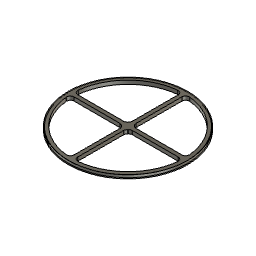
wheel v6 (Autodesk Fusion 360 design; units mm, degrees)
Autodesk Fusion 360 part; units mm, degrees
sketch "Sketch1" plane through (0, 0, 0) normal (0, 0, 1) x (1, 0, 0)
  circle A0 centre (0, 0) radius 41.275
  circle A1 centre (0, 0) radius 38.735
  circle A2 centre (0, 0) radius 3.175
  dimension "d1" = 82.55
  dimension "d2" = 77.47
  dimension "d5" = 6.35
  constraint coincident A0.centre A1.centre
  measures "d1" diameter of A0
  measures "d2" diameter of A1
  measures "d5" diameter of A2
extrude "Extrude1" add sketch "Sketch1" along normal blind 2.54 makes body 1 at (41.2237, -2.0574, 1.6933) makes body 2 at (3.1711, -0.1583, 1.6933)
sketch "Sketch4" plane through (0, 0, 0) normal (0, 0, 1) x (1, 0, 0)
  line L0 (-1.27, 39.37) -> (1.27, 39.37)
  line L1 (1.27, 39.37) -> (1.27, 1.27)
  line L2 (1.27, 1.27) -> (-1.27, 1.27)
  line L3 (-1.27, 1.27) -> (-1.27, 39.37)
  dimension "d12" = 2.54
  dimension "d13" = 1.27
  dimension "d14" = 38.1
  dimension "d15" = 1.27
  constraint horizontal L0
  constraint vertical L1
  constraint horizontal L2
  constraint vertical L3
  measures "d12" distance of L1.end L2.end
  measures "d13" horizontal distance of origin L1.end
  measures "d14" distance of L0.end L1.end
  measures "d15" vertical distance of origin L2.end
extrude "Extrude3" add sketch "Sketch4" along normal blind 2.54 separate body makes body 3
pattern_circular "C-Pattern1" count 4 over 360 about axis through (0, 0, 1.75) along (0, 0, 1) of bodies 3 makes body 4 at (-26.67, 1.27, 0.8467) makes body 5 at (-1.27, -26.67, 0.8467) makes body 6 at (26.67, -1.27, 0.8467)
combine "Combine1" operation add target body 3 tool bodies 1 2 6 5 4
fillet "Fillet1" radius 2.54 8 edges at (2.9099, 1.27, 1.27) (1.27, 2.9099, 1.27) (-1.27, 2.9099, 1.27) (-2.9099, 1.27, 1.27) (-2.9099, -1.27, 1.27) (-1.27, -2.9099, 1.27) (1.27, -2.9099, 1.27) (2.9099, -1.27, 1.27) on bodies 3
fillet "Fillet2" radius 2.54 8 edges at (1.27, -38.7142, 1.27) (-1.27, -38.7142, 1.27) (-38.7142, -1.27, 1.27) (-38.7142, 1.27, 1.27) (-1.27, 38.7142, 1.27) (1.27, 38.7142, 1.27) (38.7142, 1.27, 1.27) (38.7142, -1.27, 1.27) on bodies 3
sketch "Sketch5" plane through (0, 0, 0) normal (1, 0, 0) x (0, 1, 0)
  line L0 (-41.275, 2.54) -> (-40.8209, 2.159)
  line L1 (-40.8209, 2.159) -> (-40.8209, 0.381)
  line L2 (-40.8209, 0.381) -> (-41.275, 0)
  line L3 (-41.275, 2.54) -> (-41.275, 0)
  dimension "d24" = 1.778
  dimension "d25" = 2.54
  dimension "d26" = 130
  dimension "d27" = 130
  dimension "d28" = 41.275
  constraint vertical L1
  constraint vertical L3
  constraint horizontal origin L2.end
  measures "d24" distance of L0.end L1.end
  measures "d25" distance of L0.start L2.end
  measures "d26" angle of L0 L1
  measures "d27" angle of L1 L2
  measures "d28" horizontal distance of origin L2.end
revolve "Revolve1" cut sketch "Sketch5" angle 360 about axis through (0, 0, 1.75) along (0, 0, 1) bodies 3
fillet "Fillet3" [suppressed]
